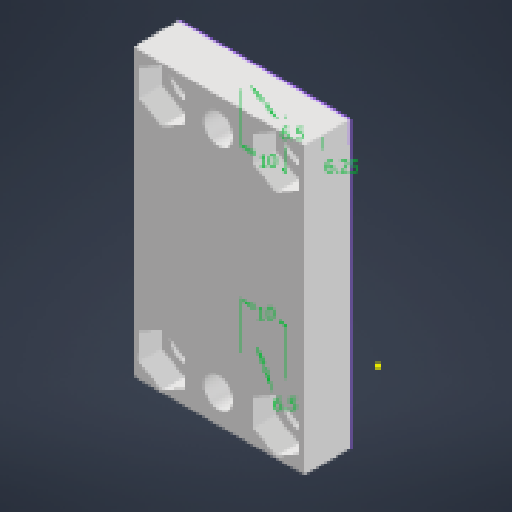
# Autodesk Inventor part: print_head_mount
Saved by Autodesk Inventor 2027 (Build 310192060, 192F)
## iProperties
Created: 2026-06-05
Part Number: print_head_mount
Material: Generic
Document SubType Name: Modeling
Designer: jacob
Density: 1 g/cm^3
Appearance: Default
Author: jacob
Autodesk Inventor part; units mm, degrees
ref_plane "YZ Plane" through (0, 0, 0) normal (1, 0, 0) x (0, 1, 0)
ref_plane "XZ Plane" through (0, 0, 0) normal (0, 1, 0) x (-1, 0, 0)
ref_plane "XY Plane" through (0, 0, 0) normal (0, 0, 1) x (1, 0, 0)
sketch "Sketch1" plane through (0, 0, 0) normal (0, 0, 1) x (1, 0, 0)
  line L0 (-6.25, 43.75) -> (-43.75, 43.75)
  line L1 (-43.75, 43.75) -> (-43.75, -18.75)
  line L2 (-43.75, -18.75) -> (-6.25, -18.75)
  line L3 (-6.25, -18.75) -> (-6.25, 43.75)
  circle A0 centre (-12.5, 37.5) radius 3.25
  circle A1 centre (-37.5, 37.5) radius 3.25
  circle A2 centre (-37.5, -12.5) radius 3.25
  line L4 (-12.5, 37.5) -> (-6.25, 37.5)
  line L5 (-12.5, -12.5) -> (-12.5, -18.75)
  line L6 (-37.5, 37.5) -> (-37.5, 43.75)
  line L7 (-37.5, -12.5) -> (-43.75, -12.5)
  circle A3 centre (-12.5, -12.5) radius 3.25
  circle A4 centre (-25.1179, 37.5) radius 3.25
  circle A5 centre (-25.1179, -12.5) radius 3.25
  line L8 (-25.1179, 31.7265) -> (-30.1179, 34.6132)
  line L9 (-30.1179, 34.6132) -> (-30.1179, 40.3868)
  line L10 (-30.1179, 40.3868) -> (-25.1179, 43.2735)
  line L11 (-25.1179, 43.2735) -> (-20.1179, 40.3868)
  line L12 (-20.1179, 40.3868) -> (-20.1179, 34.6132)
  line L13 (-20.1179, 34.6132) -> (-25.1179, 31.7265)
  line L14 (-25.1179, -6.7265) -> (-20.1179, -9.6132)
  line L15 (-20.1179, -9.6132) -> (-20.1179, -15.3868)
  line L16 (-20.1179, -15.3868) -> (-25.1179, -18.2735)
  line L17 (-25.1179, -18.2735) -> (-30.1179, -15.3868)
  line L18 (-30.1179, -15.3868) -> (-30.1179, -9.6132)
  line L19 (-30.1179, -9.6132) -> (-25.1179, -6.7265)
  point P0 (0, 0)
  point P1 (-20.1179, 37.5)
  point P2 (-30.1179, 37.5)
  point P3 (-20.1179, -12.5)
  point P4 (-30.1179, -12.5)
  dimension "d1" = 6.25
  dimension "d42" = 6.5
  dimension "d43" = 6.5
  dimension "d44" = 10
  dimension "d45" = 10
  constraints: 40 end point, 6 centre point, 4 coincident, 4 midpoint, 4 perpendicular, 4 point on line, 2 equal length, 2 parallel, 1 horizontal, 26 other
  measures "d1" distance of L4.start L4.end
  measures "d42" diameter of A4
  measures "d43" diameter of A5
  measures "d44" distance of point (-20.118, 37.5) point (-30.118, 37.5)
  measures "d45" distance of point (-20.118, -12.5) point (-30.118, -12.5)
extrude "Extrusion1" add sketch "Sketch1" along normal blind 10 contours L3 L2 L1 L0 | L8 L9 L10 L11 L12 L13 | L14 L15 L16 L17 L18 L19
sketch "Sketch2" plane through (0, 0, 10) normal (0, 0, 1) x (1, 0, 0)
  circle A0 centre (-12.5, 37.5) radius 3.25 projected
  circle A1 centre (-37.5, 37.5) radius 3.25 projected
  circle A2 centre (-37.5, -12.5) radius 3.25 projected
  circle A3 centre (-12.5, -12.5) radius 3.25 projected
  line L0 (-12.5, 31.7265) -> (-17.5, 34.6132)
  line L1 (-17.5, 34.6132) -> (-17.5, 40.3868)
  line L2 (-17.5, 40.3868) -> (-12.5, 43.2735)
  line L3 (-12.5, 43.2735) -> (-7.5, 40.3868)
  line L4 (-7.5, 40.3868) -> (-7.5, 34.6132)
  line L5 (-7.5, 34.6132) -> (-12.5, 31.7265)
  line L6 (-37.5, 31.7265) -> (-42.5, 34.6132)
  line L7 (-42.5, 34.6132) -> (-42.5, 40.3868)
  line L8 (-42.5, 40.3868) -> (-37.5, 43.2735)
  line L9 (-37.5, 43.2735) -> (-32.5, 40.3868)
  line L10 (-32.5, 40.3868) -> (-32.5, 34.6132)
  line L11 (-32.5, 34.6132) -> (-37.5, 31.7265)
  line L12 (-32.5208, -15.4225) -> (-37.5413, -18.2734)
  line L13 (-37.5413, -18.2734) -> (-42.5205, -15.3509)
  line L14 (-42.5205, -15.3509) -> (-42.4792, -9.5775)
  line L15 (-42.4792, -9.5775) -> (-37.4587, -6.7266)
  line L16 (-37.4587, -6.7266) -> (-32.4795, -9.6491)
  line L17 (-32.4795, -9.6491) -> (-32.5208, -15.4225)
  line L18 (-12.5, -6.7265) -> (-7.5, -9.6132)
  line L19 (-7.5, -9.6132) -> (-7.5, -15.3868)
  line L20 (-7.5, -15.3868) -> (-12.5, -18.2735)
  line L21 (-12.5, -18.2735) -> (-17.5, -15.3868)
  line L22 (-17.5, -15.3868) -> (-17.5, -9.6132)
  line L23 (-17.5, -9.6132) -> (-12.5, -6.7265)
  dimension "d33" = 10
  dimension "d34" = 10
  dimension "d35" = 10
  dimension "d36" = 10
  constraints: 48 end point, 4 coincident, 52 other
  measures "d33" distance between parallel lines of L1 L4
  measures "d34" distance between parallel lines of L22 L19
  measures "d35" distance between parallel lines of L14 L17
  measures "d36" distance between parallel lines of L7 L10
extrude "Extrusion2" cut sketch "Sketch2" against normal blind 5
extrude "Extrusion5" cut sketch "Sketch1" along normal blind 5 contours L8 L9 L10 L11 L12 L13 | L14 L15 L16 L17 L18 L19
body "Solid1"
